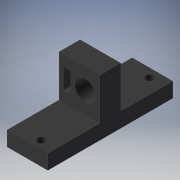
# Autodesk Inventor part: zthreadedrod
Saved by Autodesk Inventor 2019.1 (Build 231200000, 200)
## iProperties
Created: 2019-08-09
Part Number: zthreadedrod
Material: Generic
Document SubType Name: Modeling
Designer: rob
Density: 1 g/cm^3
Appearance: Default
Author: rob
Autodesk Inventor part; units mm, degrees
ref_plane "YZ Plane" through (0, 0, 0) normal (1, 0, 0) x (0, 1, 0)
ref_plane "XZ Plane" through (0, 0, 0) normal (0, 1, 0) x (-1, 0, 0)
ref_plane "XY Plane" through (0, 0, 0) normal (0, 0, 1) x (1, 0, 0)
sketch "Sketch1" plane through (0, 0, 0) normal (0, 1, 0) x (-1, 0, 0)
  line L0 (0, 0) -> (25, 0)
  line L1 (25, 0) -> (25, -60)
  line L2 (25, -60) -> (0, -60)
  line L3 (0, -60) -> (0, 0)
  circle A0 centre (12.5, -4) radius 2
  circle A1 centre (12.5, -56) radius 2
  dimension "d0" = 25
  dimension "d1" = 60
  dimension "d2" = 4
  dimension "d3" = 4
  dimension "d4" = 52
  dimension "d5" = 4
  constraints: 8 end point, 2 centre point, 2 parallel, 1 horizontal, 1 perpendicular
  measures "d0" distance of L1.end L2.end
  measures "d1" distance of L0.end L1.end
  measures "d2" diameter of A0
  measures "d3" diameter of A1
  measures "d4" distance of A1.centre A0.centre
  measures "d5" distance from line of L2 A1.centre
extrude "Extrusion1" add sketch "Sketch1" along normal blind 7
sketch "Sketch2" plane through (0, 7, 0) normal (0, 1, 0) x (1, 0, 0)
  line L0 (-25, 60) -> (-25, 0) projected
  line L1 (-25, 25) -> (0, 25)
  line L2 (0, 25) -> (0, 35)
  line L3 (0, 35) -> (-25, 35)
  line L4 (-25, 35) -> (-25, 25)
  line L5 (0, 60) -> (-25, 60) projected
  point P0 (0, 0)
  dimension "d8" = 25
  dimension "d9" = 10
  dimension "d10" = 25
  constraints: 8 end point, 2 parallel, 1 horizontal, 1 perpendicular, 1 point on line
  measures "d8" distance of L3.end L2.end
  measures "d9" distance of L2.end L1.end
  measures "d10" distance between parallel lines of L5 L3
extrude "Extrusion2" add sketch "Sketch2" along normal blind 20
sketch "Sketch3" plane through (-25, 7, -25) normal (0, 0, 1) x (1, 0, 0)
  circle A0 centre (12.5, 10) radius 5
  line L0 (2, 15.0299) -> (5.5, 15.0299)
  line L1 (5.5, 15.0299) -> (5.5, 5.0299)
  line L2 (5.5, 5.0299) -> (2, 5.0299)
  line L3 (2, 5.0299) -> (2, 15.0299)
  line L4 (19.5, 15.0299) -> (23, 15.0299)
  line L5 (23, 15.0299) -> (23, 5.0299)
  line L6 (23, 5.0299) -> (19.5, 5.0299)
  line L7 (19.5, 5.0299) -> (19.5, 15.0299)
  line L8 (0, 0) -> (0, 20) projected
  point P0 (25, -7)
  dimension "d13" = 10
  dimension "d14" = 3.5
  dimension "d15" = 10
  dimension "d16" = 3.5
  dimension "d17" = 10
  dimension "d20" = 7
  dimension "d21" = 7
  dimension "d22" = 12.5
  constraints: 16 end point, 4 parallel, 2 horizontal, 2 perpendicular, 1 centre point
  measures "d13" diameter of A0
  measures "d14" distance of L1.end L2.end
  measures "d15" distance of L0.end L1.end
  measures "d16" distance of L5.end L6.end
  measures "d17" distance of L4.end L5.end
  measures "d20" distance from line of L7 A0.centre
  measures "d21" distance from line of L1 A0.centre
  measures "d22" distance from line of L8 A0.centre
extrude "Extrusion3" cut sketch "Sketch3" against normal blind 20
sketch "Sketch4" plane through (0, 0, 0) normal (1, 0, 0) x (0, 0, -1)
  line L0 (-8.0858, 30.1503) -> (63.6355, 30.1503)
  line L1 (63.6355, 30.1503) -> (63.6355, -9.4106)
  line L2 (63.6355, -9.4106) -> (-8.0858, -9.4106)
  line L3 (-8.0858, -9.4106) -> (-8.0858, 30.1503)
  point P0 (0, 0)
  constraints: 8 end point, 2 parallel, 1 horizontal, 1 perpendicular
extrude "Extrusion4" cut sketch "Sketch4" against normal blind 5.5
body "Solid1"
